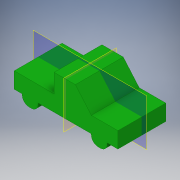
# Autodesk Inventor part: car
Saved by Autodesk Inventor 2019 (Build 230136000, 136)
## iProperties
Created: 2020-01-16
Part Number: car
Material: Generic
Document SubType Name: Modeling
Designer: tguillod
Density: 1 g/cm^3
Appearance: Dark Green
Author: tguillod
Autodesk Inventor part; units mm, degrees
ref_plane "YZ Plane" through (0, 0, 0) normal (1, 0, 0) x (0, 1, 0)
ref_plane "XZ Plane" through (0, 0, 0) normal (0, 1, 0) x (-1, 0, 0)
ref_plane "XY Plane" through (0, 0, 0) normal (0, 0, 1) x (1, 0, 0)
sketch "Sketch1" plane through (0, 0, 0) normal (0, 0, 1) x (1, 0, 0)
  line L0 (260, 0) -> (340, 0)
  line L1 (600, 260) -> (600, 340)
  line L2 (340, 600) -> (260, 600)
  line L3 (0, 340) -> (0, 260)
  line L4 (2860, 600) -> (2940, 600)
  line L5 (3200, 340) -> (3200, 260)
  line L6 (2940, 0) -> (2860, 0)
  line L7 (2600, 260) -> (2600, 340)
  arc A0 (2, 600) -> (0, 598) centre (2, 598) ccw
  arc A1 (0, 260) -> (260, 0) centre (260, 260) ccw
  arc A2 (340, 0) -> (600, 260) centre (340, 260) ccw
  arc A3 (600, 340) -> (340, 600) centre (340, 340) ccw
  arc A4 (260, 600) -> (0, 340) centre (260, 340) ccw
  arc A5 (2860, 600) -> (2600, 340) centre (2860, 340) ccw
  arc A6 (2600, 260) -> (2860, 0) centre (2860, 260) ccw
  arc A7 (2940, 0) -> (3200, 260) centre (2940, 260) ccw
  arc A8 (3200, 340) -> (2940, 600) centre (2940, 340) ccw
  point P0 (0, 0)
  point P1 (600, 600)
  point P2 (600, 0)
  point P3 (0, 600)
  point P4 (2600, 600)
  point P5 (3200, 0)
  point P6 (3200, 600)
  dimension "d0" = 600
  dimension "d1" = 600
  dimension "d2" = 600
  dimension "d3" = 2000
  dimension "d5" = 260
  constraints: 18 point on circle, 18 point on line, 18 tangent, 16 end point, 9 centre point, 7 equal radius, 4 parallel, 2 horizontal, 2 perpendicular
  measures "d0" distance of point (600, 600) point (0, 600)
  measures "d1" distance of point (600, 0) point (600, 600)
  measures "d2" distance of point (2600, 600) point (3200, 600)
  measures "d3" distance between parallel lines of L7 L1
  measures "d5" radius of A1
extrude "Extrusion1" add sketch "Sketch1" along normal blind 400
sketch "Sketch2" plane through (0, 0, 400) normal (0, 0, 1) x (1, 0, 0)
  line L0 (-300, 300) -> (3600, 300)
  line L1 (3600, 300) -> (3600, 900)
  line L2 (3600, 900) -> (2600, 900)
  line L3 (2600, 900) -> (2000, 1600)
  line L4 (2000, 1600) -> (1200, 1600)
  line L5 (1200, 1600) -> (1200, 900)
  line L6 (1200, 900) -> (-300, 900)
  line L7 (-300, 900) -> (-300, 300)
  line L8 (260, 0) -> (340, 0) projected
  line L9 (0, 340) -> (0, 260) projected
  line L10 (3200, 260) -> (3200, 340) projected
  point P0 (0, 0)
  dimension "d8" = 300
  dimension "d9" = 600
  dimension "d10" = 300
  dimension "d11" = 400
  dimension "d12" = 700
  dimension "d13" = 800
  dimension "d14" = 1000
  dimension "d15" = 1500
  constraints: 16 end point, 4 perpendicular, 2 point on line, 1 horizontal, 1 parallel
  measures "d8" distance between parallel lines of L8 L0
  measures "d9" distance of L6.end L0.start
  measures "d10" distance from line of L0.start L9
  measures "d11" distance between parallel lines of L10 L1
  measures "d12" distance of L4.end L5.end
  measures "d13" distance of L3.end L4.end
  measures "d14" distance of L1.end L2.end
  measures "d15" distance of L5.end L6.end
extrude "Extrusion2" add sketch "Sketch2" against normal blind 900
mirror "Mirror1" about plane through (1639.4502, 743.1128, -500) normal (0, 0, -1)
ref_plane "Work Plane1" through (2600, 300, -500) normal (0, 0, -1) x (-1, 0, 0)
ref_plane "Work Plane2" through (1650, 300, 400) normal (1, 0, 0) x (0, 0, -1)
body "Solid1"
